Autodesk Inventor part; units mm, degrees
(part 2 of 2)
  line L112 (37.8185, -88.0727) -> (37.0157, -88.0727)
  line L113 (37.0157, -88.0727) -> (37.0157, -81.4396)
  spline S160 degree 2 poles (33.7687, -81.3316) (34.9111, -81.3316) (36.1666, -82.6129) (36.1666, -83.7964) knots 0 0 0 1 2 2 2
  spline S161 degree 2 poles (36.1666, -83.7964) (36.1666, -84.9594) (34.9471, -86.3385) (33.9642, -86.3385) knots 0 0 0 1 2 2 2
  spline S162 degree 2 poles (33.9642, -86.3385) (33.5217, -86.3385) (32.8373, -86.0812) (32.5851, -85.8085) knots 0 0 0 1 2 2 2
  spline S163 degree 2 poles (32.5851, -85.8085) (32.3278, -85.5357) (32.0551, -84.7484) (32.0551, -84.1772) knots 0 0 0 1 2 2 2
  line L114 (32.0551, -84.1772) -> (32.0551, -83.7398)
  line L115 (32.0551, -83.7398) -> (35.3536, -83.7398)
  spline S164 degree 2 poles (35.3536, -83.7398) (35.3536, -82.9114) (34.52, -82.0314) (33.779, -82.0314) knots 0 0 0 1 2 2 2
  spline S165 degree 2 poles (33.779, -82.0314) (33.5165, -82.0314) (33.0071, -82.1498) (32.8012, -82.2424) knots 0 0 0 1 2 2 2
  spline S166 degree 2 poles (32.8012, -82.2424) (32.5851, -82.3453) (32.2867, -82.5254) (32.1889, -82.6078) knots 0 0 0 1 2 2 2
  line L116 (32.1889, -82.6078) -> (32.1426, -82.6078)
  line L117 (32.1426, -82.6078) -> (32.1426, -81.733)
  spline S167 degree 2 poles (32.1426, -81.733) (32.2815, -81.6763) (32.7035, -81.5117) (32.8681, -81.4654) knots 0 0 0 1 2 2 2
  spline S168 degree 2 poles (32.8681, -81.4654) (33.0997, -81.3985) (33.4805, -81.3316) (33.7687, -81.3316) knots 0 0 0 1 2 2 2
  spline S169 degree 2 poles (32.8373, -84.3522) (32.8476, -84.6764) (32.9814, -85.1498) (33.11, -85.3093) knots 0 0 0 1 2 2 2
  spline S170 degree 2 poles (33.11, -85.3093) (33.2489, -85.4894) (33.6863, -85.6798) (34.0105, -85.6798) knots 0 0 0 1 2 2 2
  spline S171 degree 2 poles (34.0105, -85.6798) (34.3296, -85.6798) (34.7773, -85.4894) (34.9625, -85.3042) knots 0 0 0 1 2 2 2
  spline S172 degree 2 poles (34.9625, -85.3042) (35.1426, -85.1138) (35.3279, -84.6558) (35.3536, -84.3522) knots 0 0 0 1 2 2 2
  line L118 (35.3536, -84.3522) -> (32.8373, -84.3522)
  line L119 (54.5863, -77.3087) -> (56.7733, -70.9587)
  line L120 (56.7733, -70.9587) -> (57.6841, -70.9587)
  line L121 (57.6841, -70.9587) -> (59.8711, -77.3087)
  line L122 (59.8711, -77.3087) -> (58.9654, -77.3087)
  line L123 (58.9654, -77.3087) -> (57.2055, -72.0341)
  line L124 (57.2055, -72.0341) -> (55.4456, -77.3087)
  line L125 (55.4456, -77.3087) -> (54.5863, -77.3087)
  spline S173 degree 2 poles (50.1351, -74.1337) (50.1351, -72.4252) (51.1283, -70.8249) (52.1626, -70.8249) knots 0 0 0 1 2 2 2
  spline S174 degree 2 poles (52.1626, -70.8249) (53.2123, -70.8249) (54.1952, -72.4561) (54.1952, -74.1285) knots 0 0 0 1 2 2 2
  spline S175 degree 2 poles (54.1952, -74.1285) (54.1952, -75.8472) (53.202, -77.4373) (52.1626, -77.4373) knots 0 0 0 1 2 2 2
  spline S176 degree 2 poles (52.1626, -77.4373) (51.118, -77.4373) (50.1351, -75.7906) (50.1351, -74.1337) knots 0 0 0 1 2 2 2
  spline S177 degree 2 poles (51.226, -72.1988) (51.1025, -72.5127) (50.9996, -73.4801) (50.9996, -74.1337) knots 0 0 0 1 2 2 2
  spline S178 degree 2 poles (50.9996, -74.1337) (50.9996, -74.7872) (51.1025, -75.7495) (51.2312, -76.0736) knots 0 0 0 1 2 2 2
  spline S179 degree 2 poles (51.2312, -76.0736) (51.3598, -76.3978) (51.8075, -76.7323) (52.1626, -76.7323) knots 0 0 0 1 2 2 2
  spline S180 degree 2 poles (52.1626, -76.7323) (52.5176, -76.7323) (52.9756, -76.3978) (53.1094, -76.0634) knots 0 0 0 1 2 2 2
  spline S181 degree 2 poles (53.1094, -76.0634) (53.2381, -75.7392) (53.3307, -74.7512) (53.3307, -74.1285) knots 0 0 0 1 2 2 2
  spline S182 degree 2 poles (53.3307, -74.1285) (53.3307, -73.4595) (53.2483, -72.5642) (53.1146, -72.2142) knots 0 0 0 1 2 2 2
  spline S183 degree 2 poles (53.1146, -72.2142) (52.9911, -71.8849) (52.5331, -71.5298) (52.1626, -71.5298) knots 0 0 0 1 2 2 2
  spline S184 degree 2 poles (52.1626, -71.5298) (51.8127, -71.5298) (51.3547, -71.8643) (51.226, -72.1988) knots 0 0 0 1 2 2 2
  line L126 (45.7251, -70.9587) -> (48.8229, -70.9587)
  line L127 (48.8229, -70.9587) -> (48.8229, -71.607)
  line L128 (48.8229, -71.607) -> (47.6702, -71.607)
  line L129 (47.6702, -71.607) -> (47.6702, -75.8627)
  line L130 (47.6702, -75.8627) -> (48.8229, -75.8627)
  line L131 (48.8229, -75.8627) -> (48.8229, -76.4441)
  spline S185 degree 2 poles (48.8229, -76.4441) (48.1694, -76.4441) (47.5519, -76.8147) (47.5107, -77.3292) knots 0 0 0 1 2 2 2
  line L132 (47.5107, -77.3292) -> (46.852, -77.3292)
  line L133 (46.852, -77.3292) -> (46.852, -71.607)
  line L134 (46.852, -71.607) -> (45.7251, -71.607)
  line L135 (45.7251, -71.607) -> (45.7251, -70.9587)
  point P0 (52.4636, -6.35)
  constraints: 2 end point, 2 midpoint, 1 horizontal
extrude "Extrusion14" cut sketch "Sketch15" against normal blind 3.175
equation "\"d14\" = gapBetweenParts"
equation "\"d16\" = gapBetweenParts"
equation "\"d18\" = gapBetweenParts"
equation "\"d20\" = gapBetweenParts"
equation "\"d21\" = gapBetweenParts"
equation "\"gapBetweenParts\" = 6.35"
body "Solid3"
